Autodesk Inventor part; units mm, degrees
(part 5 of 6)
  spline S209 degree 5 poles (-177.8958, 28.186) (-177.9033, 28.1852) (-177.9584, 28.1793) (-178.0614, 28.168) (-178.2121, 28.1511) (-178.4106, 28.1279) (-178.6495, 28.0989) (-178.8884, 28.0688) (-179.1273, 28.0374) (-179.3663, 28.005) (-179.6052, 27.9714) (-179.8442, 27.9367) (-180.0832, 27.9009) (-180.3222, 27.864) (-180.5612, 27.8261) (-180.8002, 27.787) (-181.0393, 27.747) (-181.2783, 27.7059) (-181.5173, 27.6638) (-181.7563, 27.6207) (-181.9952, 27.5766) (-182.2342, 27.5314) (-182.4732, 27.4854) (-182.7121, 27.4383) (-182.951, 27.3903) (-183.1899, 27.3413) (-183.4288, 27.2913) (-183.6676, 27.2405) (-183.9064, 27.1887) (-184.1452, 27.136) (-184.384, 27.0823) (-184.6227, 27.0278) (-184.8614, 26.9724) (-185.1, 26.916) (-185.3386, 26.8588) (-185.5772, 26.8007) (-185.8157, 26.7417) (-186.0542, 26.6819) (-186.2926, 26.6212) (-186.531, 26.5596) (-186.7693, 26.4972) (-187.0076, 26.434) (-187.2458, 26.3699) (-187.5316, 26.292) (-187.7697, 26.226) (-187.9601, 26.1726) (-188.1029, 26.1322) (-188.1981, 26.1051) knots 0.383497 0.383497 0.383497 0.383497 0.383497 0.383497 0.385714 0.4 0.414286 0.428571 0.442857 0.457143 0.471429 0.485714 0.5 0.514286 0.528571 0.542857 0.557143 0.571429 0.585714 0.6 0.614286 0.628571 0.642857 0.657143 0.671429 0.685714 0.7 0.714286 0.728571 0.742857 0.757143 0.771429 0.785714 0.8 0.814286 0.828571 0.842857 0.857143 0.871429 0.885714 0.9 0.914286 0.928571 0.942857 0.957143 0.971429 1 1 1 1 1 1
  arc A105 (-188.1981, 26.1051) -> (-188.7034, 22.1591) centre (0, 0) ccw
  spline S210 degree 5 poles (-179.2579, 17.5493) (-179.2649, 17.5519) (-179.3168, 17.5716) (-179.4136, 17.6085) (-179.5551, 17.6628) (-179.7414, 17.7352) (-179.9653, 17.8235) (-180.1889, 17.9129) (-180.4122, 18.0034) (-180.6353, 18.095) (-180.8581, 18.1877) (-181.0806, 18.2815) (-181.3029, 18.3764) (-181.5249, 18.4723) (-181.7466, 18.5693) (-181.9681, 18.6673) (-182.1893, 18.7662) (-182.4102, 18.8662) (-182.6309, 18.9672) (-182.8513, 19.0692) (-183.0715, 19.1721) (-183.2914, 19.2759) (-183.511, 19.3808) (-183.7304, 19.4865) (-183.9495, 19.5932) (-184.1683, 19.7008) (-184.3869, 19.8093) (-184.6052, 19.9187) (-184.8233, 20.029) (-185.0411, 20.1402) (-185.2586, 20.2523) (-185.4759, 20.3652) (-185.6929, 20.479) (-185.9096, 20.5936) (-186.1261, 20.7091) (-186.3424, 20.8255) (-186.5583, 20.9426) (-186.774, 21.0606) (-186.9894, 21.1794) (-187.2046, 21.2991) (-187.4195, 21.4195) (-187.6342, 21.5408) (-187.8486, 21.6628) (-188.1055, 21.8102) (-188.3193, 21.934) (-188.4901, 22.0337) (-188.6181, 22.1088) (-188.7034, 22.1591) knots 0.383497 0.383497 0.383497 0.383497 0.383497 0.383497 0.385714 0.4 0.414286 0.428571 0.442857 0.457143 0.471429 0.485714 0.5 0.514286 0.528571 0.542857 0.557143 0.571429 0.585714 0.6 0.614286 0.628571 0.642857 0.657143 0.671429 0.685714 0.7 0.714286 0.728571 0.742857 0.757143 0.771429 0.785714 0.8 0.814286 0.828571 0.842857 0.857143 0.871429 0.885714 0.9 0.914286 0.928571 0.942857 0.957143 0.971429 1 1 1 1 1 1
  spline S211 degree 3 poles (-178.2393, 15.9236) (-178.2044, 16.3144) (-178.4095, 17.0185) (-178.9827, 17.445) (-179.2579, 17.5493) knots 0 0 0 0 0.571429 1 1 1 1
  arc A106 (-178.2393, 15.9236) -> (-178.3666, 14.4281) centre (0, 0) ccw
  spline S212 degree 3 poles (-179.6453, 12.9979) (-179.3565, 13.0542) (-178.7193, 13.3776) (-178.3982, 14.037) (-178.3666, 14.4281) knots 0 0 0 0 0.428571 1 1 1 1
  spline S213 degree 5 poles (-179.6453, 12.9979) (-179.6526, 12.9965) (-179.7071, 12.9858) (-179.8087, 12.9659) (-179.9574, 12.9362) (-180.1533, 12.8963) (-180.3888, 12.8472) (-180.6243, 12.7969) (-180.8597, 12.7454) (-181.0951, 12.6928) (-181.3303, 12.639) (-181.5655, 12.5842) (-181.8006, 12.5283) (-182.0356, 12.4712) (-182.2706, 12.4132) (-182.5054, 12.354) (-182.7402, 12.2938) (-182.9748, 12.2326) (-183.2094, 12.1704) (-183.4439, 12.1072) (-183.6783, 12.0429) (-183.9125, 11.9777) (-184.1467, 11.9115) (-184.3808, 11.8444) (-184.6148, 11.7763) (-184.8487, 11.7072) (-185.0825, 11.6372) (-185.3161, 11.5662) (-185.5497, 11.4944) (-185.7831, 11.4216) (-186.0165, 11.3479) (-186.2497, 11.2733) (-186.4828, 11.1978) (-186.7158, 11.1215) (-186.9487, 11.0442) (-187.1815, 10.9661) (-187.4142, 10.8871) (-187.6467, 10.8073) (-187.8791, 10.7266) (-188.1114, 10.645) (-188.3436, 10.5626) (-188.5756, 10.4794) (-188.8076, 10.3953) (-189.0857, 10.2935) (-189.3174, 10.2076) (-189.5026, 10.1382) (-189.6414, 10.0858) (-189.734, 10.0507) knots 0.383497 0.383497 0.383497 0.383497 0.383497 0.383497 0.385714 0.4 0.414286 0.428571 0.442857 0.457143 0.471429 0.485714 0.5 0.514286 0.528571 0.542857 0.557143 0.571429 0.585714 0.6 0.614286 0.628571 0.642857 0.657143 0.671429 0.685714 0.7 0.714286 0.728571 0.742857 0.757143 0.771429 0.785714 0.8 0.814286 0.828571 0.842857 0.857143 0.871429 0.885714 0.9 0.914286 0.928571 0.942857 0.957143 0.971429 1 1 1 1 1 1
  arc A107 (-189.734, 10.0507) -> (-189.9028, 6.0761) centre (0, 0) ccw
  spline S214 degree 5 poles (-180.1004, 2.2839) (-180.1076, 2.286) (-180.161, 2.3012) (-180.2605, 2.3297) (-180.4062, 2.3719) (-180.5979, 2.4282) (-180.8285, 2.4971) (-181.0589, 2.5673) (-181.2891, 2.6385) (-181.5191, 2.7109) (-181.749, 2.7844) (-181.9786, 2.859) (-182.2082, 2.9346) (-182.4375, 3.0114) (-182.6666, 3.0892) (-182.8956, 3.168) (-183.1244, 3.2479) (-183.3531, 3.3288) (-183.5815, 3.4107) (-183.8098, 3.4936) (-184.0379, 3.5775) (-184.2658, 3.6623) (-184.4935, 3.7481) (-184.7211, 3.8349) (-184.9484, 3.9226) (-185.1756, 4.0113) (-185.4026, 4.1008) (-185.6294, 4.1913) (-185.856, 4.2827) (-186.0825, 4.3751) (-186.3087, 4.4683) (-186.5348, 4.5624) (-186.7607, 4.6573) (-186.9864, 4.7532) (-187.2119, 4.8499) (-187.4372, 4.9475) (-187.6623, 5.0459) (-187.8872, 5.1452) (-188.112, 5.2453) (-188.3365, 5.3463) (-188.5609, 5.4481) (-188.785, 5.5507) (-189.009, 5.6541) (-189.2775, 5.7792) (-189.501, 5.8844) (-189.6797, 5.9693) (-189.8136, 6.0332) (-189.9028, 6.0761) knots 0.383497 0.383497 0.383497 0.383497 0.383497 0.383497 0.385714 0.4 0.414286 0.428571 0.442857 0.457143 0.471429 0.485714 0.5 0.514286 0.528571 0.542857 0.557143 0.571429 0.585714 0.6 0.614286 0.628571 0.642857 0.657143 0.671429 0.685714 0.7 0.714286 0.728571 0.742857 0.757143 0.771429 0.785714 0.8 0.814286 0.828571 0.842857 0.857143 0.871429 0.885714 0.9 0.914286 0.928571 0.942857 0.957143 0.971429 1 1 1 1 1 1
  spline S215 degree 3 poles (-178.9476, 0.7504) (-178.946, 1.1428) (-179.21, 1.827) (-179.8174, 2.2033) (-180.1004, 2.2839) knots 0 0 0 0 0.571429 1 1 1 1
  arc A108 (-178.9476, 0.7504) -> (-178.9476, -0.7504) centre (0, 0) ccw
  spline S216 degree 3 poles (-180.1004, -2.2839) (-179.8174, -2.2033) (-179.21, -1.827) (-178.946, -1.1428) (-178.9476, -0.7504) knots 0 0 0 0 0.428571 1 1 1 1
  spline S217 degree 5 poles (-180.1004, -2.2839) (-180.1076, -2.286) (-180.161, -2.3012) (-180.2605, -2.3297) (-180.4062, -2.3719) (-180.5979, -2.4282) (-180.8285, -2.4971) (-181.0589, -2.5673) (-181.2891, -2.6385) (-181.5191, -2.7109) (-181.749, -2.7844) (-181.9786, -2.859) (-182.2082, -2.9346) (-182.4375, -3.0114) (-182.6666, -3.0892) (-182.8956, -3.168) (-183.1244, -3.2479) (-183.3531, -3.3288) (-183.5815, -3.4107) (-183.8098, -3.4936) (-184.0379, -3.5775) (-184.2658, -3.6623) (-184.4935, -3.7481) (-184.7211, -3.8349) (-184.9484, -3.9226) (-185.1756, -4.0113) (-185.4026, -4.1008) (-185.6294, -4.1913) (-185.856, -4.2827) (-186.0825, -4.3751) (-186.3087, -4.4683) (-186.5348, -4.5624) (-186.7607, -4.6573) (-186.9864, -4.7532) (-187.2119, -4.8499) (-187.4372, -4.9475) (-187.6623, -5.0459) (-187.8872, -5.1452) (-188.112, -5.2453) (-188.3365, -5.3463) (-188.5609, -5.4481) (-188.785, -5.5507) (-189.009, -5.6541) (-189.2775, -5.7792) (-189.501, -5.8844) (-189.6797, -5.9693) (-189.8136, -6.0332) (-189.9028, -6.0761) knots 0.383497 0.383497 0.383497 0.383497 0.383497 0.383497 0.385714 0.4 0.414286 0.428571 0.442857 0.457143 0.471429 0.485714 0.5 0.514286 0.528571 0.542857 0.557143 0.571429 0.585714 0.6 0.614286 0.628571 0.642857 0.657143 0.671429 0.685714 0.7 0.714286 0.728571 0.742857 0.757143 0.771429 0.785714 0.8 0.814286 0.828571 0.842857 0.857143 0.871429 0.885714 0.9 0.914286 0.928571 0.942857 0.957143 0.971429 1 1 1 1 1 1
  arc A109 (-189.9028, -6.0761) -> (-189.734, -10.0507) centre (0, 0) ccw
  spline S218 degree 5 poles (-179.6453, -12.9979) (-179.6526, -12.9965) (-179.7071, -12.9858) (-179.8087, -12.9659) (-179.9574, -12.9362) (-180.1533, -12.8963) (-180.3888, -12.8472) (-180.6243, -12.7969) (-180.8597, -12.7454) (-181.0951, -12.6928) (-181.3303, -12.639) (-181.5655, -12.5842) (-181.8006, -12.5283) (-182.0356, -12.4712) (-182.2706, -12.4132) (-182.5054, -12.354) (-182.7402, -12.2938) (-182.9748, -12.2326) (-183.2094, -12.1704) (-183.4439, -12.1072) (-183.6783, -12.0429) (-183.9125, -11.9777) (-184.1467, -11.9115) (-184.3808, -11.8444) (-184.6148, -11.7763) (-184.8487, -11.7072) (-185.0825, -11.6372) (-185.3161, -11.5662) (-185.5497, -11.4944) (-185.7831, -11.4216) (-186.0165, -11.3479) (-186.2497, -11.2733) (-186.4828, -11.1978) (-186.7158, -11.1215) (-186.9487, -11.0442) (-187.1815, -10.9661) (-187.4142, -10.8871) (-187.6467, -10.8073) (-187.8791, -10.7266) (-188.1114, -10.645) (-188.3436, -10.5626) (-188.5756, -10.4794) (-188.8076, -10.3953) (-189.0857, -10.2935) (-189.3174, -10.2076) (-189.5026, -10.1382) (-189.6414, -10.0858) (-189.734, -10.0507) knots 0.383497 0.383497 0.383497 0.383497 0.383497 0.383497 0.385714 0.4 0.414286 0.428571 0.442857 0.457143 0.471429 0.485714 0.5 0.514286 0.528571 0.542857 0.557143 0.571429 0.585714 0.6 0.614286 0.628571 0.642857 0.657143 0.671429 0.685714 0.7 0.714286 0.728571 0.742857 0.757143 0.771429 0.785714 0.8 0.814286 0.828571 0.842857 0.857143 0.871429 0.885714 0.9 0.914286 0.928571 0.942857 0.957143 0.971429 1 1 1 1 1 1
  spline S219 degree 3 poles (-178.3666, -14.4281) (-178.3982, -14.037) (-178.7193, -13.3776) (-179.3565, -13.0542) (-179.6453, -12.9979) knots 0 0 0 0 0.571429 1 1 1 1
  arc A110 (-178.3666, -14.4281) -> (-178.2393, -15.9236) centre (0, 0) ccw
  spline S220 degree 3 poles (-179.2579, -17.5493) (-178.9827, -17.445) (-178.4095, -17.0185) (-178.2044, -16.3144) (-178.2393, -15.9236) knots 0 0 0 0 0.428571 1 1 1 1
  spline S221 degree 5 poles (-179.2579, -17.5493) (-179.2649, -17.5519) (-179.3168, -17.5716) (-179.4136, -17.6085) (-179.5551, -17.6628) (-179.7414, -17.7352) (-179.9653, -17.8235) (-180.1889, -17.9129) (-180.4122, -18.0034) (-180.6353, -18.095) (-180.8581, -18.1877) (-181.0806, -18.2815) (-181.3029, -18.3764) (-181.5249, -18.4723) (-181.7466, -18.5693) (-181.9681, -18.6673) (-182.1893, -18.7662) (-182.4102, -18.8662) (-182.6309, -18.9672) (-182.8513, -19.0692) (-183.0715, -19.1721) (-183.2914, -19.2759) (-183.511, -19.3808) (-183.7304, -19.4865) (-183.9495, -19.5932) (-184.1683, -19.7008) (-184.3869, -19.8093) (-184.6052, -19.9187) (-184.8233, -20.029) (-185.0411, -20.1402) (-185.2586, -20.2523) (-185.4759, -20.3652) (-185.6929, -20.479) (-185.9096, -20.5936) (-186.1261, -20.7091) (-186.3424, -20.8255) (-186.5583, -20.9426) (-186.774, -21.0606) (-186.9894, -21.1794) (-187.2046, -21.2991) (-187.4195, -21.4195) (-187.6342, -21.5408) (-187.8486, -21.6628) (-188.1055, -21.8102) (-188.3193, -21.934) (-188.4901, -22.0337) (-188.6181, -22.1088) (-188.7034, -22.1591) knots 0.383497 0.383497 0.383497 0.383497 0.383497 0.383497 0.385714 0.4 0.414286 0.428571 0.442857 0.457143 0.471429 0.485714 0.5 0.514286 0.528571 0.542857 0.557143 0.571429 0.585714 0.6 0.614286 0.628571 0.642857 0.657143 0.671429 0.685714 0.7 0.714286 0.728571 0.742857 0.757143 0.771429 0.785714 0.8 0.814286 0.828571 0.842857 0.857143 0.871429 0.885714 0.9 0.914286 0.928571 0.942857 0.957143 0.971429 1 1 1 1 1 1
  arc A111 (-188.7034, -22.1591) -> (-188.1981, -26.1051) centre (0, 0) ccw
  spline S222 degree 5 poles (-177.8958, -28.186) (-177.9033, -28.1852) (-177.9584, -28.1793) (-178.0614, -28.168) (-178.2121, -28.1511) (-178.4106, -28.1279) (-178.6495, -28.0989) (-178.8884, -28.0688) (-179.1273, -28.0374) (-179.3663, -28.005) (-179.6052, -27.9714) (-179.8442, -27.9367) (-180.0832, -27.9009) (-180.3222, -27.864) (-180.5612, -27.8261) (-180.8002, -27.787) (-181.0393, -27.747) (-181.2783, -27.7059) (-181.5173, -27.6638) (-181.7563, -27.6207) (-181.9952, -27.5766) (-182.2342, -27.5314) (-182.4732, -27.4854) (-182.7121, -27.4383) (-182.951, -27.3903) (-183.1899, -27.3413) (-183.4288, -27.2913) (-183.6676, -27.2405) (-183.9064, -27.1887) (-184.1452, -27.136) (-184.384, -27.0823) (-184.6227, -27.0278) (-184.8614, -26.9724) (-185.1, -26.916) (-185.3386, -26.8588) (-185.5772, -26.8007) (-185.8157, -26.7417) (-186.0542, -26.6819) (-186.2926, -26.6212) (-186.531, -26.5596) (-186.7693, -26.4972) (-187.0076, -26.434) (-187.2458, -26.3699) (-187.5316, -26.292) (-187.7697, -26.226) (-187.9601, -26.1726) (-188.1029, -26.1322) (-188.1981, -26.1051) knots 0.383497 0.383497 0.383497 0.383497 0.383497 0.383497 0.385714 0.4 0.414286 0.428571 0.442857 0.457143 0.471429 0.485714 0.5 0.514286 0.528571 0.542857 0.557143 0.571429 0.585714 0.6 0.614286 0.628571 0.642857 0.657143 0.671429 0.685714 0.7 0.714286 0.728571 0.742857 0.757143 0.771429 0.785714 0.8 0.814286 0.828571 0.842857 0.857143 0.871429 0.885714 0.9 0.914286 0.928571 0.942857 0.957143 0.971429 1 1 1 1 1 1
  spline S223 degree 3 poles (-176.5005, -29.5027) (-176.5651, -29.1156) (-176.941, -28.4859) (-177.6033, -28.2176) (-177.8958, -28.186) knots 0 0 0 0 0.571429 1 1 1 1
  arc A112 (-176.5005, -29.5027) -> (-176.2468, -30.9819) centre (0, 0) ccw
  spline S224 degree 3 poles (-177.1239, -32.6882) (-176.8585, -32.5609) (-176.3235, -32.0874) (-176.1789, -31.3684) (-176.2468, -30.9819) knots 0 0 0 0 0.428571 1 1 1 1
  spline S225 degree 5 poles (-177.1239, -32.6882) (-177.1306, -32.6914) (-177.1806, -32.7154) (-177.2739, -32.7604) (-177.4104, -32.8265) (-177.5898, -32.9145) (-177.8054, -33.0214) (-178.0206, -33.1294) (-178.2355, -33.2386) (-178.45, -33.3488) (-178.6641, -33.4601) (-178.8779, -33.5724) (-179.0913, -33.6858) (-179.3044, -33.8002) (-179.5171, -33.9156) (-179.7294, -34.032) (-179.9415, -34.1494) (-180.1531, -34.2677) (-180.3644, -34.3871) (-180.5754, -34.5073) (-180.7861, -34.6285) (-180.9964, -34.7507) (-181.2063, -34.8738) (-181.4159, -34.9977) (-181.6252, -35.1226) (-181.8341, -35.2484) (-182.0427, -35.375) (-182.251, -35.5026) (-182.4589, -35.631) (-182.6665, -35.7602) (-182.8737, -35.8903) (-183.0806, -36.0213) (-183.2872, -36.1531) (-183.4934, -36.2857) (-183.6993, -36.4191) (-183.9049, -36.5534) (-184.1102, -36.6884) (-184.3151, -36.8243) (-184.5197, -36.961) (-184.7239, -37.0984) (-184.9279, -37.2366) (-185.1314, -37.3757) (-185.3347, -37.5154) (-185.5782, -37.6841) (-185.7807, -37.8256) (-185.9425, -37.9394) (-186.0637, -38.0251) (-186.1444, -38.0824) knots 0.383497 0.383497 0.383497 0.383497 0.383497 0.383497 0.385714 0.4 0.414286 0.428571 0.442857 0.457143 0.471429 0.485714 0.5 0.514286 0.528571 0.542857 0.557143 0.571429 0.585714 0.6 0.614286 0.628571 0.642857 0.657143 0.671429 0.685714 0.7 0.714286 0.728571 0.742857 0.757143 0.771429 0.785714 0.8 0.814286 0.828571 0.842857 0.857143 0.871429 0.885714 0.9 0.914286 0.928571 0.942857 0.957143 0.971429 1 1 1 1 1 1
  arc A113 (-186.1444, -38.0824) -> (-185.3063, -41.9713) centre (0, 0) ccw
  spline S226 degree 5 poles (-174.8646, -43.1711) (-174.8721, -43.171) (-174.9276, -43.1697) (-175.0311, -43.1672) (-175.1827, -43.1631) (-175.3824, -43.1569) (-175.6229, -43.1482) (-175.8635, -43.1384) (-176.1043, -43.1275) (-176.3451, -43.1154) (-176.5861, -43.1022) (-176.8271, -43.0879) (-177.0683, -43.0725) (-177.3096, -43.056) (-177.5509, -43.0385) (-177.7924, -43.0199) (-178.0339, -43.0002) (-178.2756, -42.9796) (-178.5173, -42.9579) (-178.7591, -42.9352) (-179.0009, -42.9115) (-179.2429, -42.8868) (-179.4849, -42.8611) (-179.727, -42.8345) (-179.9691, -42.8069) (-180.2113, -42.7784) (-180.4535, -42.7489) (-180.6958, -42.7184) (-180.9382, -42.6871) (-181.1806, -42.6548) (-181.423, -42.6216) (-181.6655, -42.5875) (-181.908, -42.5525) (-182.1506, -42.5166) (-182.3932, -42.4799) (-182.6358, -42.4422) (-182.8784, -42.4037) (-183.1211, -42.3643) (-183.3639, -42.324) (-183.6066, -42.2829) (-183.8493, -42.2409) (-184.0921, -42.1981) (-184.3349, -42.1545) (-184.6263, -42.1011) (-184.8691, -42.0556) (-185.0634, -42.0185) (-185.2091, -41.9903) (-185.3063, -41.9713) knots 0.383497 0.383497 0.383497 0.383497 0.383497 0.383497 0.385714 0.4 0.414286 0.428571 0.442857 0.457143 0.471429 0.485714 0.5 0.514286 0.528571 0.542857 0.557143 0.571429 0.585714 0.6 0.614286 0.628571 0.642857 0.657143 0.671429 0.685714 0.7 0.714286 0.728571 0.742857 0.757143 0.771429 0.785714 0.8 0.814286 0.828571 0.842857 0.857143 0.871429 0.885714 0.9 0.914286 0.928571 0.942857 0.957143 0.971429 1 1 1 1 1 1
  spline S227 degree 3 poles (-173.3626, -44.3647) (-173.4599, -43.9845) (-173.8878, -43.3889) (-174.5704, -43.1778) (-174.8646, -43.1711) knots 0 0 0 0 0.571429 1 1 1 1
  arc A114 (-173.3626, -44.3647) -> (-172.9844, -45.8171) centre (0, 0) ccw
  spline S228 degree 3 poles (-173.7136, -47.5916) (-173.46, -47.4423) (-172.9671, -46.9251) (-172.884, -46.1964) (-172.9844, -45.8171) knots 0 0 0 0 0.428571 1 1 1 1
  spline S229 degree 5 poles (-173.7136, -47.5916) (-173.7201, -47.5954) (-173.7679, -47.6235) (-173.857, -47.6762) (-173.9874, -47.7537) (-174.1587, -47.8566) (-174.3645, -47.9814) (-174.5697, -48.1073) (-174.7746, -48.2342) (-174.9789, -48.3623) (-175.1828, -48.4913) (-175.3863, -48.6213) (-175.5894, -48.7524) (-175.792, -48.8845) (-175.9941, -49.0175) (-176.1959, -49.1515) (-176.3971, -49.2864) (-176.598, -49.4223) (-176.7985, -49.5591) (-176.9985, -49.6969) (-177.1981, -49.8355) (-177.3972, -49.9751) (-177.596, -50.1155) (-177.7943, -50.2568) (-177.9923, -50.399) (-178.1898, -50.542) (-178.3869, -50.6859) (-178.5836, -50.8306) (-178.7798, -50.9762) (-178.9757, -51.1226) (-179.1712, -51.2698) (-179.3662, -51.4178) (-179.5609, -51.5667) (-179.7552, -51.7163) (-179.949, -51.8667) (-180.1425, -52.0179) (-180.3355, -52.1699) (-180.5282, -52.3226) (-180.7204, -52.4762) (-180.9123, -52.6305) (-181.1038, -52.7855) (-181.2948, -52.9413) (-181.4855, -53.0978) (-181.7138, -53.2865) (-181.9036, -53.4446) (-182.0552, -53.5718) (-182.1686, -53.6674) (-182.2442, -53.7314) knots 0.383497 0.383497 0.383497 0.383497 0.383497 0.383497 0.385714 0.4 0.414286 0.428571 0.442857 0.457143 0.471429 0.485714 0.5 0.514286 0.528571 0.542857 0.557143 0.571429 0.585714 0.6 0.614286 0.628571 0.642857 0.657143 0.671429 0.685714 0.7 0.714286 0.728571 0.742857 0.757143 0.771429 0.785714 0.8 0.814286 0.828571 0.842857 0.857143 0.871429 0.885714 0.9 0.914286 0.928571 0.942857 0.957143 0.971429 1 1 1 1 1 1
  arc A115 (-182.2442, -53.7314) -> (-181.0793, -57.5352) centre (0, 0) ccw
  spline S230 degree 5 poles (-170.5735, -57.8452) (-170.5809, -57.8456) (-170.6363, -57.8491) (-170.7397, -57.8553) (-170.8911, -57.8641) (-171.0906, -57.8749) (-171.331, -57.8867) (-171.5716, -57.8973) (-171.8124, -57.9068) (-172.0534, -57.9152) (-172.2946, -57.9225) (-172.536, -57.9287) (-172.7776, -57.9338) (-173.0194, -57.9378) (-173.2614, -57.9408) (-173.5036, -57.9427) (-173.7459, -57.9437) (-173.9884, -57.9436) (-174.2311, -57.9424) (-174.4739, -57.9403) (-174.7169, -57.9372) (-174.9601, -57.9332) (-175.2034, -57.9281) (-175.4469, -57.9221) (-175.6905, -57.9151) (-175.9342, -57.9072) (-176.1781, -57.8984) (-176.4221, -57.8886) (-176.6662, -57.8779) (-176.9105, -57.8663) (-177.1549, -57.8538) (-177.3994, -57.8404) (-177.644, -57.8261) (-177.8887, -57.8109) (-178.1335, -57.7948) (-178.3785, -57.7779) (-178.6235, -57.7601) (-178.8687, -57.7414) (-179.114, -57.7219) (-179.3593, -57.7015) (-179.6047, -57.6803) (-179.8503, -57.6582) (-180.0959, -57.6353) (-180.3908, -57.6068) (-180.6366, -57.582) (-180.8333, -57.5616) (-180.9809, -57.5458) (-181.0793, -57.5352) knots 0.383497 0.383497 0.383497 0.383497 0.383497 0.383497 0.385714 0.4 0.414286 0.428571 0.442857 0.457143 0.471429 0.485714 0.5 0.514286 0.528571 0.542857 0.557143 0.571429 0.585714 0.6 0.614286 0.628571 0.642857 0.657143 0.671429 0.685714 0.7 0.714286 0.728571 0.742857 0.757143 0.771429 0.785714 0.8 0.814286 0.828571 0.842857 0.857143 0.871429 0.885714 0.9 0.914286 0.928571 0.942857 0.957143 0.971429 1 1 1 1 1 1
  spline S231 degree 3 poles (-168.9757, -58.907) (-169.1048, -58.5365) (-169.5817, -57.9793) (-170.2798, -57.8268) (-170.5735, -57.8452) knots 0 0 0 0 0.571429 1 1 1 1
  arc A116 (-168.9757, -58.907) -> (-168.4757, -60.3221) centre (0, 0) ccw
  spline S232 degree 3 poles (-169.0518, -62.1521) (-168.8117, -61.9818) (-168.3644, -61.4246) (-168.3434, -60.6916) (-168.4757, -60.3221) knots 0 0 0 0 0.428571 1 1 1 1
  spline S233 degree 5 poles (-169.0518, -62.1521) (-169.0579, -62.1564) (-169.1031, -62.1885) (-169.1875, -62.2486) (-169.3108, -62.3369) (-169.4728, -62.4538) (-169.6672, -62.5957) (-169.8611, -62.7385) (-170.0544, -62.8824) (-170.2472, -63.0273) (-170.4394, -63.1731) (-170.6311, -63.32) (-170.8223, -63.4678) (-171.013, -63.6166) (-171.2031, -63.7663) (-171.3928, -63.9169) (-171.5819, -64.0684) (-171.7705, -64.2208) (-171.9586, -64.3742) (-172.1462, -64.5284) (-172.3334, -64.6834) (-172.52, -64.8394) (-172.7061, -64.9961) (-172.8918, -65.1538) (-173.0769, -65.3122) (-173.2616, -65.4715) (-173.4458, -65.6316) (-173.6295, -65.7925) (-173.8127, -65.9541) (-173.9955, -66.1166) (-174.1777, -66.2799) (-174.3595, -66.4439) (-174.5409, -66.6087) (-174.7217, -66.7743) (-174.9021, -66.9406) (-175.0821, -67.1077) (-175.2615, -67.2755) (-175.4405, -67.444) (-175.6191, -67.6133) (-175.7972, -67.7833) (-175.9748, -67.954) (-176.152, -68.1254) (-176.3287, -68.2975) (-176.5402, -68.5049) (-176.7159, -68.6786) (-176.8561, -68.8181) (-176.961, -68.9231) (-177.0309, -68.9932) knots 0.383497 0.383497 0.383497 0.383497 0.383497 0.383497 0.385714 0.4 0.414286 0.428571 0.442857 0.457143 0.471429 0.485714 0.5 0.514286 0.528571 0.542857 0.557143 0.571429 0.585714 0.6 0.614286 0.628571 0.642857 0.657143 0.671429 0.685714 0.7 0.714286 0.728571 0.742857 0.757143 0.771429 0.785714 0.8 0.814286 0.828571 0.842857 0.857143 0.871429 0.885714 0.9 0.914286 0.928571 0.942857 0.957143 0.971429 1 1 1 1 1 1
  arc A117 (-177.0309, -68.9932) -> (-175.5476, -72.6845) centre (0, 0) ccw
  spline S234 degree 5 poles (-165.0534, -72.1024) (-165.0608, -72.1035) (-165.1157, -72.1116) (-165.2181, -72.1267) (-165.3682, -72.1482) (-165.5662, -72.1759) (-165.8046, -72.208) (-166.0435, -72.239) (-166.2826, -72.2689) (-166.522, -72.2977) (-166.7617, -72.3254) (-167.0017, -72.3521) (-167.242, -72.3776) (-167.4826, -72.4022) (-167.7235, -72.4257) (-167.9646, -72.4481) (-168.206, -72.4696) (-168.4477, -72.4901) (-168.6896, -72.5095) (-168.9317, -72.528) (-169.1741, -72.5456) (-169.4167, -72.5621) (-169.6596, -72.5777) (-169.9027, -72.5924) (-170.146, -72.6061) (-170.3895, -72.6189) (-170.6333, -72.6308) (-170.8772, -72.6417) (-171.1214, -72.6518) (-171.3657, -72.6609) (-171.6103, -72.6692) (-171.8551, -72.6766) (-172.1, -72.683) (-172.3451, -72.6887) (-172.5905, -72.6934) (-172.836, -72.6973) (-173.0817, -72.7003) (-173.3275, -72.7025) (-173.5735, -72.7039) (-173.8197, -72.7043) (-174.0661, -72.704) (-174.3126, -72.7028) (-174.5593, -72.7009) (-174.8555, -72.6975) (-175.1025, -72.6937) (-175.3003, -72.6899) (-175.4487, -72.6868) (-175.5476, -72.6845) knots 0.383497 0.383497 0.383497 0.383497 0.383497 0.383497 0.385714 0.4 0.414286 0.428571 0.442857 0.457143 0.471429 0.485714 0.5 0.514286 0.528571 0.542857 0.557143 0.571429 0.585714 0.6 0.614286 0.628571 0.642857 0.657143 0.671429 0.685714 0.7 0.714286 0.728571 0.742857 0.757143 0.771429 0.785714 0.8 0.814286 0.828571 0.842857 0.857143 0.871429 0.885714 0.9 0.914286 0.928571 0.942857 0.957143 0.971429 1 1 1 1 1 1
  spline S235 degree 3 poles (-163.3713, -73.0249) (-163.5314, -72.6667) (-164.0538, -72.152) (-164.7623, -72.0593) (-165.0534, -72.1024) knots 0 0 0 0 0.571429 1 1 1 1
  arc A118 (-163.3713, -73.0249) -> (-162.7531, -74.3926) centre (0, 0) ccw
  spline S236 degree 3 poles (-163.1719, -76.2648) (-162.9472, -76.0748) (-162.5487, -75.4817) (-162.5899, -74.7494) (-162.7531, -74.3926) knots 0 0 0 0 0.428571 1 1 1 1
  spline S237 degree 5 poles (-163.1719, -76.2648) (-163.1776, -76.2696) (-163.22, -76.3054) (-163.2989, -76.3724) (-163.4143, -76.4708) (-163.5658, -76.6011) (-163.7475, -76.7589) (-163.9285, -76.9177) (-164.109, -77.0775) (-164.2888, -77.2382) (-164.4679, -77.3998) (-164.6465, -77.5624) (-164.8245, -77.7259) (-165.0018, -77.8903) (-165.1786, -78.0556) (-165.3548, -78.2217) (-165.5304, -78.3888) (-165.7054, -78.5566) (-165.8798, -78.7254) (-166.0537, -78.8949) (-166.227, -79.0653) (-166.3997, -79.2365) (-166.5719, -79.4085) (-166.7435, -79.5813) (-166.9145, -79.7549) (-167.085, -79.9292) (-167.255, -80.1044) (-167.4244, -80.2802) (-167.5932, -80.4569) (-167.7616, -80.6343) (-167.9293, -80.8124) (-168.0966, -80.9913) (-168.2633, -81.1709) (-168.4295, -81.3512) (-168.5951, -81.5322) (-168.7602, -81.7139) (-168.9248, -81.8963) (-169.0889, -82.0794) (-169.2524, -82.2633) (-169.4154, -82.4477) (-169.578, -82.6329) (-169.74, -82.8187) (-169.9014, -83.0052) (-170.0946, -83.2298) (-170.2549, -83.4178) (-170.3828, -83.5687) (-170.4784, -83.6821) (-170.5421, -83.7579) knots 0.383497 0.383497 0.383497 0.383497 0.383497 0.383497 0.385714 0.4 0.414286 0.428571 0.442857 0.457143 0.471429 0.485714 0.5 0.514286 0.528571 0.542857 0.557143 0.571429 0.585714 0.6 0.614286 0.628571 0.642857 0.657143 0.671429 0.685714 0.7 0.714286 0.728571 0.742857 0.757143 0.771429 0.785714 0.8 0.814286 0.828571 0.842857 0.857143 0.871429 0.885714 0.9 0.914286 0.928571 0.942857 0.957143 0.971429 1 1 1 1 1 1
  arc A119 (-170.5421, -83.7579) -> (-168.7511, -87.3102) centre (0, 0) ccw
  spline S238 degree 5 poles (-158.3441, -85.8402) (-158.3513, -85.8419) (-158.4053, -85.8546) (-158.5062, -85.8783) (-158.6539, -85.9125) (-158.8488, -85.9569) (-159.0837, -86.0091) (-159.319, -86.0602) (-159.5547, -86.1103) (-159.7908, -86.1593) (-160.0273, -86.2072) (-160.2642, -86.2541) (-160.5015, -86.3) (-160.7391, -86.3449) (-160.9771, -86.3887) (-161.2155, -86.4315) (-161.4542, -86.4734) (-161.6932, -86.5143) (-161.9326, -86.5542) (-162.1723, -86.5932) (-162.4124, -86.6312) (-162.6527, -86.6682) (-162.8934, -86.7044) (-163.1343, -86.7396) (-163.3756, -86.7739) (-163.6172, -86.8073) (-163.859, -86.8398) (-164.1012, -86.8714) (-164.3436, -86.9022) (-164.5863, -86.932) (-164.8293, -86.961) (-165.0725, -86.9891) (-165.3161, -87.0163) (-165.5598, -87.0427) (-165.8039, -87.0682) (-166.0482, -87.0929) (-166.2927, -87.1168) (-166.5375, -87.1398) (-166.7825, -87.162) (-167.0278, -87.1834) (-167.2733, -87.2039) (-167.519, -87.2237) (-167.765, -87.2426) (-168.0604, -87.2644) (-168.3069, -87.2815) (-168.5042, -87.2946) (-168.6523, -87.304) (-168.7511, -87.3102) knots 0.383497 0.383497 0.383497 0.383497 0.383497 0.383497 0.385714 0.4 0.414286 0.428571 0.442857 0.457143 0.471429 0.485714 0.5 0.514286 0.528571 0.542857 0.557143 0.571429 0.585714 0.6 0.614286 0.628571 0.642857 0.657143 0.671429 0.685714 0.7 0.714286 0.728571 0.742857 0.757143 0.771429 0.785714 0.8 0.814286 0.828571 0.842857 0.857143 0.871429 0.885714 0.9 0.914286 0.928571 0.942857 0.957143 0.971429 1 1 1 1 1 1
  spline S239 degree 3 poles (-156.5898, -86.6167) (-156.7797, -86.2734) (-157.3439, -85.8048) (-158.0577, -85.7725) (-158.3441, -85.8402) knots 0 0 0 0 0.571429 1 1 1 1
  arc A120 (-156.5898, -86.6167) -> (-155.8578, -87.927) centre (0, 0) ccw
  spline S240 degree 3 poles (-156.1164, -89.828) (-155.9086, -89.6196) (-155.5618, -88.9948) (-155.665, -88.2687) (-155.8578, -87.927) knots 0 0 0 0 0.428571 1 1 1 1
  spline S241 degree 5 poles (-156.1164, -89.828) (-156.1216, -89.8333) (-156.1608, -89.8726) (-156.2338, -89.946) (-156.3404, -90.0539) (-156.4803, -90.1965) (-156.648, -90.3692) (-156.8149, -90.5427) (-156.9811, -90.7172) (-157.1466, -90.8926) (-157.3115, -91.0689) (-157.4756, -91.246) (-157.6391, -91.424) (-157.8019, -91.6028) (-157.964, -91.7825) (-158.1254, -91.963) (-158.2862, -92.1443) (-158.4464, -92.3264) (-158.6059, -92.5094) (-158.7647, -92.693) (-158.923, -92.8775) (-159.0805, -93.0627) (-159.2375, -93.2487) (-159.3938, -93.4354) (-159.5495, -93.6229) (-159.7046, -93.8111) (-159.8591, -94) (-160.013, -94.1896) (-160.1663, -94.3799) (-160.3189, -94.571) (-160.471, -94.7627) (-160.6225, -94.9551) (-160.7733, -95.1482) (-160.9236, -95.3419) (-161.0733, -95.5363) (-161.2224, -95.7314) (-161.371, -95.9271) (-161.5189, -96.1235) (-161.6663, -96.3205) (-161.8131, -96.5181) (-161.9593, -96.7164) (-162.1049, -96.9153) (-162.25, -97.1148) (-162.4234, -97.355) (-162.5673, -97.5559) (-162.6819, -97.7171) (-162.7676, -97.8382) (-162.8246, -97.9191) knots 0.383497 0.383497 0.383497 0.383497 0.383497 0.383497 0.385714 0.4 0.414286 0.428571 0.442857 0.457143 0.471429 0.485714 0.5 0.514286 0.528571 0.542857 0.557143 0.571429 0.585714 0.6 0.614286 0.628571 0.642857 0.657143 0.671429 0.685714 0.7 0.714286 0.728571 0.742857 0.757143 0.771429 0.785714 0.8 0.814286 0.828571 0.842857 0.857143 0.871429 0.885714 0.9 0.914286 0.928571 0.942857 0.957143 0.971429 1 1 1 1 1 1
  arc A121 (-162.8246, -97.9191) -> (-160.7388, -101.3067) centre (0, 0) ccw
  spline S242 degree 5 poles (-150.4939, -98.9594) (-150.501, -98.9618) (-150.5537, -98.9791) (-150.6522, -99.0112) (-150.7965, -99.0578) (-150.9869, -99.1185) (-151.2165, -99.1905) (-151.4466, -99.2614) (-151.6772, -99.3313) (-151.9084, -99.4001) (-152.14, -99.4679) (-152.372, -99.5348) (-152.6045, -99.6006) (-152.8375, -99.6654) (-153.0709, -99.7293) (-153.3048, -99.7922) (-153.5391, -99.8541) (-153.7738, -99.9152) (-154.009, -99.9752) (-154.2445, -100.0344) (-154.4804, -100.0926) (-154.7168, -100.1499) (-154.9535, -100.2064) (-155.1906, -100.2619) (-155.4281, -100.3165) (-155.666, -100.3703) (-155.9042, -100.4232) (-156.1428, -100.4752) (-156.3817, -100.5264) (-156.621, -100.5767) (-156.8607, -100.6262) (-157.1007, -100.6748) (-157.341, -100.7226) (-157.5817, -100.7696) (-157.8227, -100.8157) (-158.064, -100.861) (-158.3056, -100.9056) (-158.5476, -100.9492) (-158.7898, -100.9921) (-159.0324, -101.0342) (-159.2753, -101.0755) (-159.5184, -101.1161) (-159.7619, -101.1558) (-160.0544, -101.2025) (-160.2985, -101.2405) (-160.4941, -101.2703) (-160.6409, -101.2922) (-160.7388, -101.3067) knots 0.383497 0.383497 0.383497 0.383497 0.383497 0.383497 0.385714 0.4 0.414286 0.428571 0.442857 0.457143 0.471429 0.485714 0.5 0.514286 0.528571 0.542857 0.557143 0.571429 0.585714 0.6 0.614286 0.628571 0.642857 0.657143 0.671429 0.685714 0.7 0.714286 0.728571 0.742857 0.757143 0.771429 0.785714 0.8 0.814286 0.828571 0.842857 0.857143 0.871429 0.885714 0.9 0.914286 0.928571 0.942857 0.957143 0.971429 1 1 1 1 1 1
  spline S243 degree 3 poles (-148.6801, -99.5844) (-148.8984, -99.2584) (-149.5003, -98.8394) (-150.2143, -98.8677) (-150.4939, -98.9594) knots 0 0 0 0 0.571429 1 1 1 1
  arc A122 (-148.6801, -99.5844) -> (-147.8396, -100.8279) centre (0, 0) ccw
  spline S244 degree 3 poles (-147.936, -102.744) (-147.7466, -102.5187) (-147.4541, -101.8668) (-147.6185, -101.1521) (-147.8396, -100.8279) knots 0 0 0 0 0.428571 1 1 1 1
  spline S245 degree 5 poles (-147.936, -102.744) (-147.9408, -102.7497) (-147.9765, -102.7921) (-148.043, -102.8715) (-148.1401, -102.988) (-148.2674, -103.1421) (-148.4198, -103.3283) (-148.5714, -103.5154) (-148.7222, -103.7033) (-148.8723, -103.8921) (-149.0216, -104.0817) (-149.1701, -104.2721) (-149.3179, -104.4634) (-149.4649, -104.6554) (-149.6112, -104.8481) (-149.7568, -105.0417) (-149.9016, -105.236) (-150.0457, -105.431) (-150.1892, -105.6268) (-150.3319, -105.8233) (-150.4739, -106.0205) (-150.6152, -106.2184) (-150.7558, -106.4171) (-150.8957, -106.6164) (-151.035, -106.8164) (-151.1736, -107.017) (-151.3115, -107.2184) (-151.4487, -107.4203) (-151.5853, -107.623) (-151.7212, -107.8263) (-151.8565, -108.0302) (-151.9911, -108.2347) (-152.125, -108.4399) (-152.2583, -108.6457) (-152.391, -108.8521) (-152.523, -109.0591) (-152.6544, -109.2668) (-152.7852, -109.475) (-152.9153, -109.6838) (-153.0448, -109.8931) (-153.1737, -110.1031) (-153.302, -110.3136) (-153.4296, -110.5247) (-153.582, -110.7787) (-153.7083, -110.9911) (-153.8088, -111.1614) (-153.8839, -111.2894) (-153.9339, -111.3749) knots 0.383497 0.383497 0.383497 0.383497 0.383497 0.383497 0.385714 0.4 0.414286 0.428571 0.442857 0.457143 0.471429 0.485714 0.5 0.514286 0.528571 0.542857 0.557143 0.571429 0.585714 0.6 0.614286 0.628571 0.642857 0.657143 0.671429 0.685714 0.7 0.714286 0.728571 0.742857 0.757143 0.771429 0.785714 0.8 0.814286 0.828571 0.842857 0.857143 0.871429 0.885714 0.9 0.914286 0.928571 0.942857 0.957143 0.971429 1 1 1 1 1 1
  arc A123 (-153.9339, -111.3749) -> (-151.5683, -114.5734) centre (0, 0) ccw
  spline S246 degree 5 poles (-141.5594, -111.3657) (-141.5662, -111.3686) (-141.6173, -111.3903) (-141.7127, -111.4307) (-141.8525, -111.4894) (-142.0371, -111.566) (-142.2598, -111.6572) (-142.4831, -111.7474) (-142.7069, -111.8366) (-142.9314, -111.9248) (-143.1564, -112.012) (-143.382, -112.0982) (-143.6081, -112.1835) (-143.8347, -112.2679) (-144.0619, -112.3513) (-144.2896, -112.4339) (-144.5178, -112.5154) (-144.7465, -112.5961) (-144.9756, -112.6759) (-145.2053, -112.7549) (-145.4355, -112.8329) (-145.6661, -112.91) (-145.8972, -112.9863) (-146.1287, -113.0618) (-146.3607, -113.1364) (-146.5932, -113.2101) (-146.8261, -113.283) (-147.0594, -113.3551) (-147.2931, -113.4263) (-147.5273, -113.4968) (-147.7619, -113.5664) (-147.9969, -113.6352) (-148.2323, -113.7032) (-148.4681, -113.7704) (-148.7043, -113.8368) (-148.9409, -113.9025) (-149.1779, -113.9673) (-149.4153, -114.0314) (-149.6531, -114.0946) (-149.8912, -114.1572) (-150.1297, -114.2189) (-150.3685, -114.2799) (-150.6078, -114.3401) (-150.8953, -114.4115) (-151.1353, -114.47) (-151.3276, -114.5163) (-151.472, -114.5506) (-151.5683, -114.5734) knots 0.383497 0.383497 0.383497 0.383497 0.383497 0.383497 0.385714 0.4 0.414286 0.428571 0.442857 0.457143 0.471429 0.485714 0.5 0.514286 0.528571 0.542857 0.557143 0.571429 0.585714 0.6 0.614286 0.628571 0.642857 0.657143 0.671429 0.685714 0.7 0.714286 0.728571 0.742857 0.757143 0.771429 0.785714 0.8 0.814286 0.828571 0.842857 0.857143 0.871429 0.885714 0.9 0.914286 0.928571 0.942857 0.957143 0.971429 1 1 1 1 1 1
  spline S247 degree 3 poles (-139.6991, -111.8346) (-139.9443, -111.5283) (-140.5796, -111.1618) (-141.2886, -111.2506) (-141.5594, -111.3657) knots 0 0 0 0 0.571429 1 1 1 1
  arc A124 (-139.6991, -111.8346) -> (-138.7562, -113.0023) centre (0, 0) ccw
  spline S248 degree 3 poles (-138.6898, -114.9197) (-138.5202, -114.6792) (-138.284, -114.0048) (-138.5084, -113.3066) (-138.7562, -113.0023) knots 0 0 0 0 0.428571 1 1 1 1
  spline S249 degree 5 poles (-138.6898, -114.9197) (-138.6941, -114.9258) (-138.726, -114.9711) (-138.7856, -115.0558) (-138.8724, -115.1802) (-138.9862, -115.3445) (-139.1223, -115.5429) (-139.2575, -115.7422) (-139.3918, -115.9423) (-139.5253, -116.1431) (-139.658, -116.3447) (-139.7898, -116.547) (-139.9209, -116.7501) (-140.0511, -116.9538) (-140.1805, -117.1583) (-140.3091, -117.3635) (-140.437, -117.5694) (-140.564, -117.776) (-140.6903, -117.9832) (-140.8158, -118.1911) (-140.9406, -118.3997) (-141.0646, -118.6088) (-141.1879, -118.8187) (-141.3104, -119.0291) (-141.4322, -119.2402) (-141.5533, -119.4519) (-141.6736, -119.6642) (-141.7932, -119.8771) (-141.9121, -120.0906) (-142.0303, -120.3047) (-142.1478, -120.5193) (-142.2646, -120.7346) (-142.3806, -120.9504) (-142.496, -121.1667) (-142.6107, -121.3836) (-142.7247, -121.6011) (-142.838, -121.8191) (-142.9507, -122.0377) (-143.0626, -122.2568) (-143.1739, -122.4764) (-143.2845, -122.6965) (-143.3944, -122.9171) (-143.5037, -123.1383) (-143.6341, -123.4043) (-143.7419, -123.6266) (-143.8276, -123.8049) (-143.8916, -123.9388) (-143.9341, -124.0281) knots 0.383497 0.383497 0.383497 0.383497 0.383497 0.383497 0.385714 0.4 0.414286 0.428571 0.442857 0.457143 0.471429 0.485714 0.5 0.514286 0.528571 0.542857 0.557143 0.571429 0.585714 0.6 0.614286 0.628571 0.642857 0.657143 0.671429 0.685714 0.7 0.714286 0.728571 0.742857 0.757143 0.771429 0.785714 0.8 0.814286 0.828571 0.842857 0.857143 0.871429 0.885714 0.9 0.914286 0.928571 0.942857 0.957143 0.971429 1 1 1 1 1 1
  arc A125 (-143.9341, -124.0281) -> (-141.3058, -127.0145) centre (0, 0) ccw
  spline S250 degree 5 poles (-131.6049, -122.9696) (-131.6115, -122.9731) (-131.6606, -122.999) (-131.7522, -123.0473) (-131.8865, -123.1177) (-132.0639, -123.2097) (-132.2781, -123.3194) (-132.4929, -123.4282) (-132.7084, -123.5361) (-132.9246, -123.643) (-133.1414, -123.749) (-133.3588, -123.854) (-133.5769, -123.9582) (-133.7956, -124.0615) (-134.0148, -124.1639) (-134.2347, -124.2654) (-134.4552, -124.3661) (-134.6762, -124.4659) (-134.8978, -124.5648) (-135.1199, -124.6629) (-135.3426, -124.7602) (-135.5659, -124.8566) (-135.7897, -124.9523) (-136.014, -125.0471) (-136.2388, -125.1411) (-136.4642, -125.2342) (-136.6901, -125.3266) (-136.9164, -125.4182) (-137.1433, -125.5091) (-137.3706, -125.5991) (-137.5985, -125.6884) (-137.8268, -125.7768) (-138.0556, -125.8646) (-138.2849, -125.9515) (-138.5146, -126.0377) (-138.7448, -126.1232) (-138.9754, -126.2079) (-139.2065, -126.2919) (-139.438, -126.3751) (-139.67, -126.4576) (-139.9024, -126.5393) (-140.1352, -126.6203) (-140.3685, -126.7006) (-140.6489, -126.7961) (-140.8831, -126.8748) (-141.0708, -126.9372) (-141.2117, -126.9837) (-141.3058, -127.0145) knots 0.383497 0.383497 0.383497 0.383497 0.383497 0.383497 0.385714 0.4 0.414286 0.428571 0.442857 0.457143 0.471429 0.485714 0.5 0.514286 0.528571 0.542857 0.557143 0.571429 0.585714 0.6 0.614286 0.628571 0.642857 0.657143 0.671429 0.685714 0.7 0.714286 0.728571 0.742857 0.757143 0.771429 0.785714 0.8 0.814286 0.828571 0.842857 0.857143 0.871429 0.885714 0.9 0.914286 0.928571 0.942857 0.957143 0.971429 1 1 1 1 1 1
  spline S251 degree 3 poles (-129.7116, -123.279) (-129.9819, -122.9946) (-130.646, -122.6833) (-131.3448, -122.8319) (-131.6049, -122.9696) knots 0 0 0 0 0.571429 1 1 1 1
  arc A126 (-129.7116, -123.279) -> (-128.6731, -124.3626) centre (0, 0) ccw
  spline S252 degree 3 poles (-128.4443, -126.2674) (-128.2957, -126.0134) (-128.1176, -125.3214) (-128.4004, -124.6447) (-128.6731, -124.3626) knots 0 0 0 0 0.428571 1 1 1 1
  spline S253 degree 5 poles (-128.4443, -126.2674) (-128.448, -126.2738) (-128.476, -126.3217) (-128.5282, -126.4112) (-128.6042, -126.5424) (-128.7036, -126.7158) (-128.8224, -126.9251) (-128.9402, -127.1351) (-129.0571, -127.3458) (-129.173, -127.5573) (-129.2881, -127.7694) (-129.4024, -127.9821) (-129.5157, -128.1956) (-129.6282, -128.4097) (-129.7398, -128.6244) (-129.8505, -128.8398) (-129.9605, -129.0558) (-130.0695, -129.2724) (-130.1778, -129.4895) (-130.2852, -129.7073) (-130.3919, -129.9257) (-130.4977, -130.1447) (-130.6027, -130.3642) (-130.707, -130.5843) (-130.8104, -130.8049) (-130.9131, -131.0261) (-131.015, -131.2479) (-131.1161, -131.4702) (-131.2165, -131.693) (-131.3161, -131.9163) (-131.415, -132.1401) (-131.5131, -132.3645) (-131.6104, -132.5894) (-131.707, -132.8147) (-131.8029, -133.0406) (-131.898, -133.2669) (-131.9925, -133.4938) (-132.0862, -133.7211) (-132.1791, -133.9489) (-132.2714, -134.1771) (-132.3629, -134.4059) (-132.4538, -134.635) (-132.5439, -134.8647) (-132.6512, -135.1408) (-132.7398, -135.3714) (-132.81, -135.5563) (-132.8624, -135.6951) (-132.8972, -135.7878) knots 0.383497 0.383497 0.383497 0.383497 0.383497 0.383497 0.385714 0.4 0.414286 0.428571 0.442857 0.457143 0.471429 0.485714 0.5 0.514286 0.528571 0.542857 0.557143 0.571429 0.585714 0.6 0.614286 0.628571 0.642857 0.657143 0.671429 0.685714 0.7 0.714286 0.728571 0.742857 0.757143 0.771429 0.785714 0.8 0.814286 0.828571 0.842857 0.857143 0.871429 0.885714 0.9 0.914286 0.928571 0.942857 0.957143 0.971429 1 1 1 1 1 1
  arc A127 (-132.8972, -135.7878) -> (-130.0251, -138.5405) centre (0, 0) ccw
  spline S254 degree 5 poles (-120.7023, -133.6875) (-120.7086, -133.6915) (-120.7552, -133.7215) (-120.8424, -133.7774) (-120.9703, -133.8589) (-121.1393, -133.9656) (-121.3433, -134.0931) (-121.5482, -134.2197) (-121.7538, -134.3455) (-121.9601, -134.4703) (-122.1671, -134.5943) (-122.3748, -134.7175) (-122.5833, -134.8398) (-122.7924, -134.9612) (-123.0022, -135.0818) (-123.2127, -135.2016) (-123.4238, -135.3206) (-123.6356, -135.4388) (-123.848, -135.5562) (-124.061, -135.6728) (-124.2747, -135.7886) (-124.4889, -135.9036) (-124.7038, -136.0179) (-124.9193, -136.1314) (-125.1353, -136.2441) (-125.352, -136.3561) (-125.5692, -136.4673) (-125.787, -136.5777) (-126.0053, -136.6875) (-126.2242, -136.7965) (-126.4437, -136.9047) (-126.6637, -137.0123) (-126.8842, -137.1191) (-127.1053, -137.2252) (-127.3268, -137.3305) (-127.5489, -137.4352) (-127.7716, -137.5392) (-127.9947, -137.6424) (-128.2183, -137.745) (-128.4425, -137.8468) (-128.6671, -137.948) (-128.8922, -138.0485) (-129.1178, -138.1483) (-129.3891, -138.2672) (-129.6158, -138.3655) (-129.7975, -138.4435) (-129.934, -138.5018) (-130.0251, -138.5405) knots 0.383497 0.383497 0.383497 0.383497 0.383497 0.383497 0.385714 0.4 0.414286 0.428571 0.442857 0.457143 0.471429 0.485714 0.5 0.514286 0.528571 0.542857 0.557143 0.571429 0.585714 0.6 0.614286 0.628571 0.642857 0.657143 0.671429 0.685714 0.7 0.714286 0.728571 0.742857 0.757143 0.771429 0.785714 0.8 0.814286 0.828571 0.842857 0.857143 0.871429 0.885714 0.9 0.914286 0.928571 0.942857 0.957143 0.971429 1 1 1 1 1 1
  spline S255 degree 3 poles (-118.7895, -133.8352) (-119.083, -133.5748) (-119.771, -133.3209) (-120.4548, -133.5282) (-120.7023, -133.6875) knots 0 0 0 0 0.571429 1 1 1 1
  arc A128 (-118.7895, -133.8352) -> (-117.6628, -134.8268) centre (0, 0) ccw
  spline S256 degree 3 poles (-117.2733, -136.7053) (-117.1468, -136.4396) (-117.028, -135.7351) (-117.3672, -135.0848) (-117.6628, -134.8268) knots 0 0 0 0 0.428571 1 1 1 1
  spline S257 degree 5 poles (-117.2733, -136.7053) (-117.2765, -136.7121) (-117.3004, -136.7622) (-117.3447, -136.8558) (-117.4093, -136.993) (-117.4937, -137.1741) (-117.5943, -137.3927) (-117.6938, -137.612) (-117.7924, -137.8319) (-117.8901, -138.0524) (-117.9868, -138.2735) (-118.0825, -138.4952) (-118.1774, -138.7175) (-118.2713, -138.9403) (-118.3643, -139.1637) (-118.4564, -139.3877) (-118.5476, -139.6122) (-118.6379, -139.8373) (-118.7274, -140.0629) (-118.8159, -140.289) (-118.9037, -140.5157) (-118.9906, -140.7428) (-119.0766, -140.9705) (-119.1618, -141.1986) (-119.2462, -141.4272) (-119.3297, -141.6563) (-119.4124, -141.8859) (-119.4943, -142.116) (-119.5754, -142.3465) (-119.6558, -142.5774) (-119.7353, -142.8089) (-119.814, -143.0407) (-119.8919, -143.2731) (-119.9691, -143.5058) (-120.0454, -143.739) (-120.1211, -143.9726) (-120.1959, -144.2066) (-120.27, -144.441) (-120.3433, -144.6759) (-120.4159, -144.9112) (-120.4877, -145.1468) (-120.5587, -145.3829) (-120.6291, -145.6193) (-120.7126, -145.9035) (-120.7813, -146.1409) (-120.8356, -146.331) (-120.876, -146.4738) (-120.9029, -146.5691) knots 0.383497 0.383497 0.383497 0.383497 0.383497 0.383497 0.385714 0.4 0.414286 0.428571 0.442857 0.457143 0.471429 0.485714 0.5 0.514286 0.528571 0.542857 0.557143 0.571429 0.585714 0.6 0.614286 0.628571 0.642857 0.657143 0.671429 0.685714 0.7 0.714286 0.728571 0.742857 0.757143 0.771429 0.785714 0.8 0.814286 0.828571 0.842857 0.857143 0.871429 0.885714 0.9 0.914286 0.928571 0.942857 0.957143 0.971429 1 1 1 1 1 1
  arc A129 (-120.9029, -146.5691) -> (-117.8077, -149.0683) centre (0, 0) ccw
  spline S258 degree 5 poles (-108.93, -143.4421) (-108.9359, -143.4467) (-108.9798, -143.4806) (-109.062, -143.5436) (-109.1825, -143.6357) (-109.3418, -143.7563) (-109.5343, -143.9007) (-109.7277, -144.0442) (-109.9219, -144.1869) (-110.1168, -144.3288) (-110.3126, -144.47) (-110.5091, -144.6103) (-110.7065, -144.7498) (-110.9045, -144.8885) (-111.1033, -145.0265) (-111.3029, -145.1637) (-111.5032, -145.3002) (-111.7042, -145.4359) (-111.9058, -145.5709) (-112.1082, -145.7051) (-112.3113, -145.8386) (-112.515, -145.9714) (-112.7194, -146.1035) (-112.9245, -146.2348) (-113.1302, -146.3655) (-113.3366, -146.4954) (-113.5436, -146.6247) (-113.7512, -146.7532) (-113.9595, -146.8811) (-114.1683, -147.0082) (-114.3778, -147.1347) (-114.5879, -147.2605) (-114.7986, -147.3856) (-115.0098, -147.5101) (-115.2217, -147.6339) (-115.4341, -147.757) (-115.6471, -147.8795) (-115.8607, -148.0013) (-116.0748, -148.1224) (-116.2895, -148.2429) (-116.5048, -148.3628) (-116.7206, -148.482) (-116.9369, -148.6006) (-117.1971, -148.7421) (-117.4146, -148.8592) (-117.5891, -148.9524) (-117.7202, -149.022) (-117.8077, -149.0683) knots 0.383497 0.383497 0.383497 0.383497 0.383497 0.383497 0.385714 0.4 0.414286 0.428571 0.442857 0.457143 0.471429 0.485714 0.5 0.514286 0.528571 0.542857 0.557143 0.571429 0.585714 0.6 0.614286 0.628571 0.642857 0.657143 0.671429 0.685714 0.7 0.714286 0.728571 0.742857 0.757143 0.771429 0.785714 0.8 0.814286 0.828571 0.842857 0.857143 0.871429 0.885714 0.9 0.914286 0.928571 0.942857 0.957143 0.971429 1 1 1 1 1 1
  spline S259 degree 3 poles (-107.0115, -143.4271) (-107.326, -143.1925) (-108.0331, -142.9979) (-108.6969, -143.2625) (-108.93, -143.4421) knots 0 0 0 0 0.571429 1 1 1 1
  arc A130 (-107.0115, -143.4271) -> (-105.8048, -144.3196) centre (0, 0) ccw
  spline S260 degree 3 poles (-105.2574, -146.1583) (-105.1539, -145.8829) (-105.0953, -145.1707) (-105.4884, -144.5516) (-105.8048, -144.3196) knots 0 0 0 0 0.428571 1 1 1 1
  spline S261 degree 5 poles (-105.2574, -146.1583) (-105.26, -146.1653) (-105.2796, -146.2173) (-105.3158, -146.3143) (-105.3685, -146.4565) (-105.4373, -146.6441) (-105.5189, -146.8705) (-105.5995, -147.0974) (-105.6791, -147.3248) (-105.7577, -147.5528) (-105.8353, -147.7813) (-105.9119, -148.0103) (-105.9876, -148.2399) (-106.0622, -148.4699) (-106.1359, -148.7004) (-106.2087, -148.9314) (-106.2806, -149.1628) (-106.3515, -149.3947) (-106.4215, -149.6271) (-106.4906, -149.8599) (-106.5588, -150.0932) (-106.6261, -150.3269) (-106.6925, -150.561) (-106.758, -150.7955) (-106.8227, -151.0305) (-106.8865, -151.2659) (-106.9495, -151.5016) (-107.0116, -151.7378) (-107.0728, -151.9744) (-107.1333, -152.2113) (-107.1929, -152.4487) (-107.2516, -152.6864) (-107.3096, -152.9245) (-107.3667, -153.1629) (-107.4231, -153.4017) (-107.4786, -153.6409) (-107.5333, -153.8804) (-107.5872, -154.1203) (-107.6404, -154.3605) (-107.6927, -154.6011) (-107.7443, -154.842) (-107.7951, -155.0832) (-107.8451, -155.3248) (-107.9042, -155.6151) (-107.9525, -155.8573) (-107.9906, -156.0514) (-108.0187, -156.1971) (-108.0374, -156.2944) knots 0.383497 0.383497 0.383497 0.383497 0.383497 0.383497 0.385714 0.4 0.414286 0.428571 0.442857 0.457143 0.471429 0.485714 0.5 0.514286 0.528571 0.542857 0.557143 0.571429 0.585714 0.6 0.614286 0.628571 0.642857 0.657143 0.671429 0.685714 0.7 0.714286 0.728571 0.742857 0.757143 0.771429 0.785714 0.8 0.814286 0.828571 0.842857 0.857143 0.871429 0.885714 0.9 0.914286 0.928571 0.942857 0.957143 0.971429 1 1 1 1 1 1
  arc A131 (-108.0374, -156.2944) -> (-104.7414, -158.5221) centre (0, 0) ccw
  spline S262 degree 5 poles (-96.3728, -152.1633) (-96.3783, -152.1683) (-96.4192, -152.2058) (-96.4957, -152.2756) (-96.608, -152.3776) (-96.7565, -152.5113) (-96.9361, -152.6715) (-97.1166, -152.8309) (-97.298, -152.9895) (-97.4802, -153.1475) (-97.6633, -153.3047) (-97.8472, -153.4611) (-98.032, -153.6169) (-98.2176, -153.7719) (-98.404, -153.9263) (-98.5912, -154.0799) (-98.7792, -154.2329) (-98.9679, -154.3852) (-99.1574, -154.5368) (-99.3477, -154.6877) (-99.5387, -154.8379) (-99.7304, -154.9875) (-99.9229, -155.1364) (-100.1161, -155.2847) (-100.31, -155.4323) (-100.5046, -155.5793) (-100.6999, -155.7256) (-100.8959, -155.8713) (-101.0926, -156.0164) (-101.2899, -156.1608) (-101.4879, -156.3046) (-101.6865, -156.4477) (-101.8858, -156.5903) (-102.0858, -156.7322) (-102.2864, -156.8735) (-102.4876, -157.0142) (-102.6895, -157.1543) (-102.8919, -157.2938) (-103.095, -157.4326) (-103.2987, -157.5709) (-103.503, -157.7086) (-103.7079, -157.8457) (-103.9134, -157.9822) (-104.1607, -158.1452) (-104.3675, -158.2804) (-104.5334, -158.388) (-104.6581, -158.4685) (-104.7414, -158.5221) knots 0.383497 0.383497 0.383497 0.383497 0.383497 0.383497 0.385714 0.4 0.414286 0.428571 0.442857 0.457143 0.471429 0.485714 0.5 0.514286 0.528571 0.542857 0.557143 0.571429 0.585714 0.6 0.614286 0.628571 0.642857 0.657143 0.671429 0.685714 0.7 0.714286 0.728571 0.742857 0.757143 0.771429 0.785714 0.8 0.814286 0.828571 0.842857 0.857143 0.871429 0.885714 0.9 0.914286 0.928571 0.942857 0.957143 0.971429 1 1 1 1 1 1
  spline S263 degree 3 poles (-94.4626, -151.9857) (-94.7958, -151.7785) (-95.5169, -151.6446) (-96.1558, -151.9645) (-96.3728, -152.1633) knots 0 0 0 0 0.571429 1 1 1 1
  arc A132 (-94.4626, -151.9857) -> (-93.1845, -152.7726) centre (0, 0) ccw
  spline S264 degree 3 poles (-92.4831, -154.5582) (-92.4034, -154.275) (-92.4054, -153.5605) (-92.8495, -152.9769) (-93.1845, -152.7726) knots 0 0 0 0 0.428571 1 1 1 1